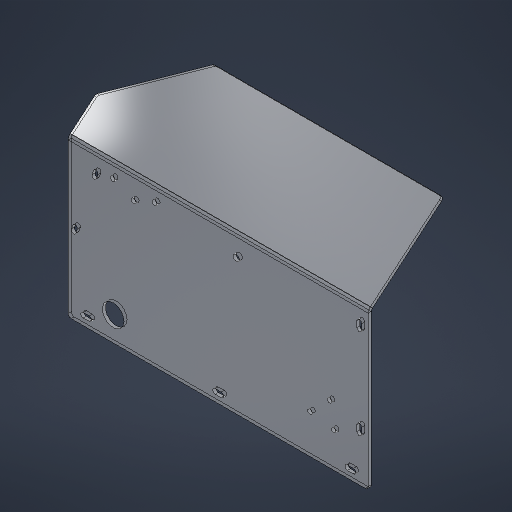
# Autodesk Inventor part: TURRET,WIRE,PLATE,BOTTOM
Saved by Autodesk Inventor 2026.1 (Build 301233020, 233B)
## iProperties
Created: 2026-03-17
Part Number: TURRET,WIRE,PLATE,BOTTOM
Material: Polycarbonate, Clear
Document SubType Name: Sheet Metal
Designer: Owen L
Density: 1.2 g/cm^3
Flat Pattern Width: 26.4768 cm
Flat Pattern Length: 31.75 cm
Flat Pattern Area: 840.637 cm^2
Sheet Metal Rule: Default
Sheet Metal Width: 10.424 in
Sheet Metal Length: 12.500 in
Sheet Metal Area: 130.299 in^2
Appearance: Polycarbonate - Clear
Mass: 307.775 g
Surface Area: 1663.25 cm^2
Volume: 256.479 cm^3
Author: Owen L
Autodesk Inventor part; units mm, degrees
ref_plane "YZ Plane" through (0, 0, 0) normal (1, 0, 0) x (0, 1, 0)
ref_plane "XZ Plane" through (0, 0, 0) normal (0, 1, 0) x (-1, 0, 0)
ref_plane "XY Plane" through (0, 0, 0) normal (0, 0, 1) x (1, 0, 0)
sketch "Sketch1" plane through (0, 0, 0) normal (0, 0, 1) x (1, 0, 0)
  arc A0 (-3.175, 3.175) -> (0, 0) centre (0, 3.175) ccw
  line L0 (0, 0) -> (311.15, 0)
  arc A1 (311.15, 0) -> (314.325, 3.175) centre (311.15, 3.175) ccw
  line L1 (314.325, 3.175) -> (314.325, 161.925)
  line L2 (311.15, 165.1) -> (12.1553, 165.1)
  line L3 (-3.175, 149.7697) -> (-3.175, 3.175)
  line L4 (292.1, 12.065) -> (298.45, 12.065)
  arc A2 (298.45, 6.985) -> (298.45, 12.065) centre (298.45, 9.525) ccw
  line L5 (298.45, 6.985) -> (292.1, 6.985)
  arc A3 (292.1, 12.065) -> (292.1, 6.985) centre (292.1, 9.525) ccw
  line L6 (302.26, 47.625) -> (302.26, 53.975)
  arc A4 (307.34, 53.975) -> (302.26, 53.975) centre (304.8, 53.975) ccw
  line L7 (307.34, 53.975) -> (307.34, 47.625)
  arc A5 (302.26, 47.625) -> (307.34, 47.625) centre (304.8, 47.625) ccw
  line L8 (152.4, 12.065) -> (158.75, 12.065)
  arc A6 (158.75, 6.985) -> (158.75, 12.065) centre (158.75, 9.525) ccw
  line L9 (158.75, 6.985) -> (152.4, 6.985)
  arc A7 (152.4, 12.065) -> (152.4, 6.985) centre (152.4, 9.525) ccw
  line L10 (12.7, 12.065) -> (19.05, 12.065)
  arc A8 (19.05, 6.985) -> (19.05, 12.065) centre (19.05, 9.525) ccw
  line L11 (19.05, 6.985) -> (12.7, 6.985)
  arc A9 (12.7, 12.065) -> (12.7, 6.985) centre (12.7, 9.525) ccw
  line L12 (302.26, 142.875) -> (302.26, 149.225)
  arc A10 (307.34, 149.225) -> (302.26, 149.225) centre (304.8, 149.225) ccw
  line L13 (307.34, 149.225) -> (307.34, 142.875)
  arc A11 (302.26, 142.875) -> (307.34, 142.875) centre (304.8, 142.875) ccw
  line L14 (0.2503, 82.1064) -> (1.9189, 86.7699)
  arc A12 (6.4628, 85.1441) -> (1.9189, 86.7699) centre (4.1909, 85.957) ccw
  line L15 (6.4628, 85.1441) -> (4.7942, 80.4806)
  arc A13 (0.2503, 82.1064) -> (4.7942, 80.4806) centre (2.5223, 81.2935) ccw
  line L16 (28.2458, 146.0235) -> (26.5772, 141.36)
  arc A14 (22.0333, 142.9859) -> (26.5772, 141.36) centre (24.3053, 142.1729) ccw
  line L17 (22.0333, 142.9859) -> (23.702, 147.6493)
  arc A15 (28.2458, 146.0235) -> (23.702, 147.6493) centre (25.9739, 146.8364) ccw
  circle A16 centre (88.302, 150.3688) radius 2.5797
  circle A17 centre (66.077, 140.8438) radius 2.5797
  circle A18 centre (43.852, 150.3688) radius 2.5797
  circle A19 centre (273.2565, 61.6719) radius 2.413
  circle A20 centre (252.6531, 41.0685) radius 2.413
  circle A21 centre (277.6672, 36.6578) radius 2.413
  circle A22 centre (44.45, 25.4) radius 11.43
  line L18 (12.1553, 165.1) -> (-3.175, 165.1)
  line L19 (-3.175, 165.1) -> (-3.175, 149.7697)
  line L20 (314.325, 161.925) -> (314.325, 165.1)
  line L21 (314.325, 165.1) -> (311.15, 165.1)
  point P0 (0, 0)
  point P1 (-3.175, 3.175)
  point P2 (0, 0)
  point P3 (314.325, 3.175)
  point P4 (22.0333, 142.9859)
  point P5 (23.702, 147.6493)
  point P6 (28.2458, 146.0235)
  point P7 (26.5772, 141.36)
  point P8 (6.4628, 85.1441)
  point P9 (19.05, 6.985)
  point P10 (158.75, 6.985)
  point P11 (298.45, 6.985)
  dimension "GapSize" = 3.175
extrude "Plate1" add sketch "Sketch1" along normal blind 3.175
sketch "Sketch2" plane through (314.325, 162.6678, 1.1341) normal (0, 0.7660444, 0.6427876) x (-1, 0, 0)
  line L0 (317.5, 0) -> (0, 0)
  line L1 (0, 0) -> (0, -101.6)
  line L2 (0, -101.6) -> (317.5, -101.6)
  line L3 (317.5, -101.6) -> (317.5, 0)
  constraints: 6 end point, 1 horizontal, 1 perpendicular, 1 vertical
edge flange "Flange1" height 101.6 angle 50 thickness 3.175 bend radius 3.175 thickness toward (0, 0.7660444, 0.6427876) relief tear relief width 3.175 relief depth 1.5875 edges at (161.6526, 165.1, 0) wall of the first edge with corners at (-3.175, 162.6678, 1.1341) (314.325, 162.6678, 1.1341) (314.325, 227.975, -76.696) (-3.175, 227.975, -76.696)
bend "Bend1"
corner "Corner1"
chamfer "Corner Chamfer1" distance 76.2 distance2 63.5 1 edges at (-3.175, 229.1911, -75.6755) measured on face at (102.6583, 228.7858, -76.0157)
sketch "Sketch3" plane through (0, 0, 3.175) normal (0, 0, 1) x (1, 0, 0)
  line L0 (311.15, 0) -> (0, 0) projected
  line L1 (-3.175, 3.175) -> (-3.175, 162.1389) projected
  point P0 (174.625, 142.875)
  dimension "d149" = 142.875
  dimension "d150" = 177.8
  measures "d149" distance from line of L0 point (174.625, 142.875)
  measures "d150" distance from line of L1 point (174.625, 142.875)
hole "Hole1" at (174.625, 142.875, 3.175) direction (0, 0, -1) diameter 6.604 end through all
fillet "Corner Round1" radius 3.175 3 edges at (314.325, 229.1911, -75.6755) (73.025, 229.1911, -75.6755) (-3.175, 188.3741, -27.0317)
equation "\"GapSize\" = Thickness"
equation "\"d156\" = Thickness"
equation "\"d135\" = Thickness"
equation "\"d136\" = BendReliefWidth"
equation "\"d137\" = BendReliefDepth"
equation "\"d138\" = MinimumRemnant"
equation "\"d139\" = TransitionRadius"
equation "\"d142\" = BendRadius"
equation "\"d143\" = CornerReliefSize"
equation "\"d144\" = GapSize"
equation "\"d145\" = JacobiRadiusSize"
equation "\"BendRadius\" = Thickness"
equation "\"BendReliefWidth\" = Thickness"
equation "\"BendReliefDepth\" = 0.5 * Thickness"
equation "\"CornerReliefSize\" = 4 * Thickness"
equation "\"MinimumRemnant\" = 2 * Thickness"
equation "\"TransitionRadius\" = BendRadius"
equation "\"JacobiRadiusSize\" = BendRadius"
equation "\"Thickness\" = 3.175"
body "Solid1"
